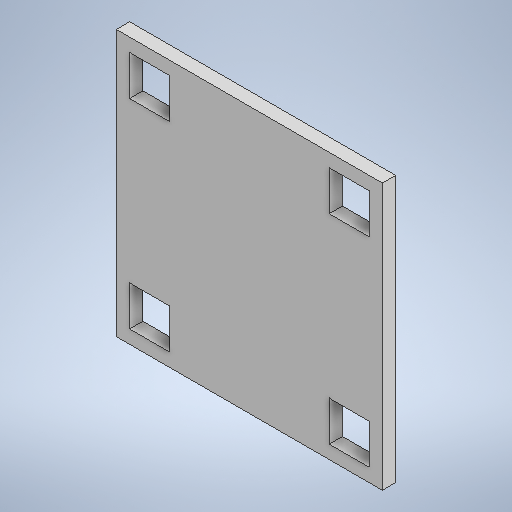
# Autodesk Inventor part: Base
Saved by Autodesk Inventor 2026 (Build 300175050, 175E)
## iProperties
Created: 2025-04-13
Part Number: Base
Material: Genérico
Document SubType Name: Modeling
Designer: piero
Density: 1 g/cm^3
Appearance: Valor por defecto
Author: piero
Autodesk Inventor part; units mm, degrees
ref_plane "YZ Plane" through (0, 0, 0) normal (1, 0, 0) x (0, 1, 0)
ref_plane "XZ Plane" through (0, 0, 0) normal (0, 1, 0) x (-1, 0, 0)
ref_plane "XY Plane" through (0, 0, 0) normal (0, 0, 1) x (1, 0, 0)
sketch "Boceto1" plane through (0, 0, 0) normal (0, 0, 1) x (1, 0, 0)
  line L0 (0, 0) -> (1000, 0)
  line L1 (1000, 0) -> (1000, 1000)
  line L2 (1000, 1000) -> (0, 1000)
  line L3 (0, 1000) -> (0, 0)
  dimension "d0" = 1000
  dimension "d1" = 1000
  constraints: 8 end point, 2 parallel, 1 horizontal, 1 perpendicular
  measures "d0" distance of L1.end L2.end
  measures "d1" distance of L0.end L1.end
extrude "Extrusión1" add sketch "Boceto1" along normal blind 50
sketch "Boceto3" plane through (0, 0, 50) normal (0, 0, 1) x (1, 0, 0)
  line L0 (1000, 1000) -> (0, 1000) projected
  line L1 (0, 1000) -> (0, 0) projected
  line L2 (50, 950) -> (200, 950)
  line L3 (200, 950) -> (200, 800)
  line L4 (200, 800) -> (50, 800)
  line L5 (50, 800) -> (50, 950)
  line L6 (800, 800) -> (950, 800)
  line L7 (950, 800) -> (950, 950)
  line L8 (950, 950) -> (800, 950)
  line L9 (800, 950) -> (800, 800)
  line L10 (800, 800) -> (950, 950) construction
  line L11 (950, 800) -> (800, 950) construction
  line L12 (1000, 0) -> (1000, 1000) projected
  line L13 (850, 900) -> (900, 900)
  line L14 (900, 900) -> (900, 850)
  line L15 (900, 850) -> (850, 850)
  line L16 (850, 850) -> (850, 900)
  line L17 (850, 900) -> (900, 850) construction
  line L18 (900, 900) -> (850, 850) construction
  line L19 (50, 50) -> (200, 50)
  line L20 (200, 50) -> (200, 200)
  line L21 (200, 200) -> (50, 200)
  line L22 (50, 200) -> (50, 50)
  line L23 (50, 50) -> (200, 200) construction
  line L24 (200, 50) -> (50, 200) construction
  line L25 (0, 0) -> (1000, 0) projected
  line L26 (100, 100) -> (150, 100)
  line L27 (150, 100) -> (150, 150)
  line L28 (150, 150) -> (100, 150)
  line L29 (100, 150) -> (100, 100)
  line L30 (100, 100) -> (150, 150) construction
  line L31 (150, 100) -> (100, 150) construction
  line L32 (800, 50) -> (950, 50)
  line L33 (950, 50) -> (950, 200)
  line L34 (950, 200) -> (800, 200)
  line L35 (800, 200) -> (800, 50)
  line L36 (800, 50) -> (950, 200) construction
  line L37 (950, 50) -> (800, 200) construction
  line L38 (850, 150) -> (900, 150)
  line L39 (900, 150) -> (900, 100)
  line L40 (900, 100) -> (850, 100)
  line L41 (850, 100) -> (850, 150)
  line L42 (850, 150) -> (900, 100) construction
  line L43 (900, 150) -> (850, 100) construction
  line L44 (50, 450) -> (200, 600) construction
  line L45 (200, 450) -> (50, 600) construction
  line L46 (100, 550) -> (150, 500) construction
  line L47 (150, 550) -> (100, 500) construction
  line L48 (100, 900) -> (150, 900)
  line L49 (150, 900) -> (150, 850)
  line L50 (150, 850) -> (100, 850)
  line L51 (100, 850) -> (100, 900)
  line L52 (100, 900) -> (150, 850) construction
  line L53 (150, 900) -> (100, 850) construction
  point P0 (875, 875)
  point P1 (125, 125)
  point P2 (875, 125)
  point P3 (875, 125)
  point P4 (125, 525)
  point P5 (125, 525)
  point P6 (125, 875)
  point P7 (125, 900)
  point P8 (125, 950)
  point P9 (50, 875)
  dimension "d19" = 150
  dimension "d20" = 150
  dimension "d21" = 50
  dimension "d22" = 50
  dimension "d25" = 150
  dimension "d26" = 150
  dimension "d27" = 50
  dimension "d28" = 50
  dimension "d29" = 50
  dimension "d30" = 50
  dimension "d31" = 150
  dimension "d32" = 150
  dimension "d33" = 50
  dimension "d34" = 50
  dimension "d35" = 50
  dimension "d36" = 50
  dimension "d37" = 150
  dimension "d38" = 150
  dimension "d39" = 50
  dimension "d40" = 50
  dimension "d41" = 50
  dimension "d42" = 50
  dimension "d43" = 150
  dimension "d44" = 150
  dimension "d45" = 50
  dimension "d46" = 50
  dimension "d48" = 400
  dimension "d51" = 50
  dimension "d52" = 50
  dimension "d53" = 50
  dimension "d54" = 50
  constraints: 100 end point, 23 midpoint, 16 parallel, 8 horizontal, 8 perpendicular
  measures "d19" distance of L3.end L4.end
  measures "d20" distance of L2.end L3.end
  measures "d21" distance between parallel lines of L2 L0
  measures "d22" distance between parallel lines of L5 L1
  measures "d25" distance of L8.end L7.end
  measures "d26" distance of L7.end L6.end
  measures "d27" distance between parallel lines of L8 L0
  measures "d28" distance between parallel lines of L7 L12
  measures "d29" distance of L14.end L15.end
  measures "d30" distance of L13.end L14.end
  measures "d31" distance of L21.end L20.end
  measures "d32" distance of L20.end L19.end
  measures "d33" distance between parallel lines of L1 L22
  measures "d34" distance between parallel lines of L19 L25
  measures "d35" distance of L28.end L27.end
  measures "d36" distance of L27.end L26.end
  measures "d37" distance of L34.end L33.end
  measures "d38" distance of L33.end L32.end
  measures "d39" distance of L39.end L40.end
  measures "d40" distance of L38.end L39.end
  measures "d41" distance between parallel lines of L12 L33
  measures "d42" distance between parallel lines of L25 L32
  measures "d43" distance of L45.end L44.end
  measures "d44" distance of L44.end L45.start
  measures "d45" distance of L46.end L47.end
  measures "d46" distance of L47.start L46.end
  measures "d48" distance of point (125, 525) point (125, 125)
  measures "d51" distance of L49.end L50.end
  measures "d52" distance of L48.end L49.end
  measures "d53" distance of point (125, 900) point (125, 950)
  measures "d54" distance from line of point (50, 875) L51
extrude "Extrusión2" cut sketch "Boceto3" against normal blind 50 contours L2 L3 L4 L5 | L9 L8 L7 L6 | L13 L14 L15 L16 | L22 L21 L20 L19 | L29 L28 L27 L26 | L35 L34 L33 L32 | L38 L39 L40 L41 | L48 L49 L50 L51
